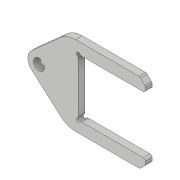
# Autodesk Inventor part: FRC003-1
Saved by Autodesk Inventor 2020 (Build 240168000, 168)
## iProperties
Created: 2020-02-07
Part Number: FRC003-1
Material: Generic
Document SubType Name: Modeling
Designer: Juan Carlos Botero
Density: 1 g/cm^3
Appearance: Default
Mass: 6.52409 g
Surface Area: 32.0611 cm^2
Volume: 6.52409 cm^3
Author: Juan Carlos Botero
Title: SOPORTE PIVOTE
Autodesk Inventor part; units mm, degrees
ref_plane "YZ Plane" through (0, 0, 0) normal (1, 0, 0) x (0, 1, 0)
ref_plane "XZ Plane" through (0, 0, 0) normal (0, 1, 0) x (-1, 0, 0)
ref_plane "XY Plane" through (0, 0, 0) normal (0, 0, 1) x (1, 0, 0)
sketch "Sketch1" plane through (0, 0, 0) normal (0, 0, 1) x (1, 0, 0)
  circle A0 centre (-790.1228, -10.9134) radius 9.525 projected
  ellipse E0 centre (61.5218, 18.65) end of major axis (52.5416, 18.65) minor radius 6.35 (61.5218, 25) -> (52.5416, 18.65) ccw
  line L0 (61.5218, 25) -> (114.272, 25)
  ellipse E1 centre (114.272, 18.65) end of major axis (105.2917, 18.65) minor radius 6.35 (123.2522, 18.65) -> (114.272, 25) ccw
  line L1 (123.2522, 18.65) -> (123.2522, -18.65)
  ellipse E2 centre (114.272, -18.65) end of major axis (105.2917, -18.65) minor radius 6.35 (114.272, -25) -> (123.2522, -18.65) ccw
  line L2 (114.272, -25) -> (61.5218, -25)
  ellipse E3 centre (61.5218, -18.65) end of major axis (52.5416, -18.65) minor radius 6.35 (52.5416, -18.65) -> (61.5218, -25) ccw
  line L3 (52.5416, -18.65) -> (52.5416, 18.65)
  line L4 (114.272, 21.825) -> (61.5218, 21.825)
  ellipse E4 centre (61.5218, 18.65) end of major axis (57.0317, 18.65) minor radius 3.175 (61.5218, 21.825) -> (57.0317, 18.65) ccw
  line L5 (57.0317, 18.65) -> (57.0317, -18.65)
  ellipse E5 centre (61.5218, -18.65) end of major axis (57.0317, -18.65) minor radius 3.175 (57.0317, -18.65) -> (61.5218, -21.825) ccw
  line L6 (61.5218, -21.825) -> (114.272, -21.825)
  ellipse E6 centre (114.272, -18.65) end of major axis (109.7818, -18.65) minor radius 3.175 (114.272, -21.825) -> (118.7621, -18.65) ccw
  line L7 (118.7621, -18.65) -> (118.7621, 18.65)
  ellipse E7 centre (114.272, 18.65) end of major axis (109.7818, 18.65) minor radius 3.175 (118.7621, 18.65) -> (114.272, 21.825) ccw
  circle A1 centre (17.6912, 0) radius 5 projected
  circle A2 centre (17.6912, 0) radius 10
  line L8 (15.357, 9.7238) -> (52.5416, 18.65)
  line L9 (52.5416, -18.65) -> (15.357, -9.7238)
  dimension "d4" = 20
  constraints: 20 end point, 4 horizontal, 4 vertical, 2 point on circle, 2 tangent, 1 centre point, 1 coincident, 56 other
  measures "d4" diameter of A2
extrude "Extrusion1" add sketch "Sketch1" along normal blind 6 contours L3 L9 A2 L8 | A2
chamfer "Chamfer1" distance 5 angle 45 1 edges at (52.5416, 0, 6)
thicken "Thicken1" operation add thickness 3 both sides no extend neighbours yes toward (-0.7071068, 0, -0.7071068) faces at (50.8749, 5.8166, 2.6667)
sketch "Sketch2" plane through (0, 0, 0) normal (0, 0, -1) x (-1, 0, 0)
  line L0 (-49.2989, -17.8716) -> (-49.2989, 17.8716) projected
  line L1 (-15.357, -9.7238) -> (-49.2989, -17.8716) projected
  arc A0 (-15.357, -9.7238) -> (-15.357, 9.7238) centre (-17.6912, 0) ccw projected
  line L2 (-49.2989, 17.8716) -> (-15.357, 9.7238) projected
  circle A1 centre (-17.6912, 0) radius 5 projected
  line L3 (-112.6912, -35.5) -> (-42.6912, -35.5)
  line L4 (-42.6912, -35.5) -> (-42.6912, 35.5)
  line L5 (-42.6912, 35.5) -> (-112.6912, 35.5)
  line L6 (-112.6912, -35.5) -> (-42.6912, 35.5) construction
  line L7 (-42.6912, -35.5) -> (-112.6912, 35.5) construction
  line L8 (-42.6912, 35.5) -> (-11.061, 7.486)
  arc A2 (-15.357, -9.7238) -> (-15.357, 9.7238) centre (-17.6912, 0) ccw projected
  line L9 (-42.6912, -35.5) -> (-11.061, -7.486)
  line L10 (-102.6912, -25.5) -> (-52.6912, -25.5)
  line L11 (-52.6912, -25.5) -> (-52.6912, 25.5)
  line L12 (-52.6912, 25.5) -> (-102.6912, 25.5)
  line L13 (-102.6912, -25.5) -> (-52.6912, 25.5) construction
  line L14 (-52.6912, -25.5) -> (-102.6912, 25.5) construction
  line L15 (-102.6912, 25.5) -> (-112.6912, 25.5)
  line L16 (-112.6912, -25.5) -> (-102.6912, -25.5)
  line L17 (-112.6912, 35.5) -> (-112.6912, 25.5)
  line L18 (-112.6912, -25.5) -> (-112.6912, -35.5)
  line L19 (-49.2989, -17.8716) -> (-49.2989, 17.8716) projected
  point P0 (0, 0)
  point P1 (-77.6912, 0)
  point P2 (-49.2989, 0)
  point P3 (-77.6912, 0)
  point P4 (-11.061, -7.486)
  point P5 (-11.061, 7.486)
  point P6 (-49.2989, 0)
  point P7 (-52.6912, 0)
  dimension "d13" = 51
  dimension "d14" = 35
  dimension "d15" = 10
  dimension "d16" = 50
  dimension "d17" = 10
  dimension "d30" = 71
  constraints: 32 end point, 8 midpoint, 3 horizontal, 2 horizontal alignment, 2 parallel, 2 perpendicular, 2 point on circle, 2 tangent, 2 vertical, 1 collinear, 1 vertical alignment
  measures "d13" distance of L11.end L10.end
  measures "d14" distance from line of A0.centre L11
  measures "d15" distance between parallel lines of L12 L5
  measures "d16" distance of L11.end L12.end
  measures "d17" distance between parallel lines of L4 L11
  measures "d30" distance between parallel lines of L3 L5
extrude "Extrusion2" add sketch "Sketch2" against normal up to surface (6 mm away)
chamfer "Chamfer2" distance 5 angle 45 2 edges at (112.6912, 35.5, 3) (112.6912, -35.5, 3)
sketch "Sketch3" plane through (0, 0, 0) normal (0, 0, -1) x (-1, 0, 0)
  line L0 (-107.6912, -35.5) -> (-112.6912, -30.5) projected
  line L1 (-107.6912, -35.5) -> (-42.6912, -35.5) projected
  line L2 (-42.6912, -35.5) -> (-11.061, -7.486) projected
  arc A0 (-11.061, -7.486) -> (-11.061, 7.486) centre (-17.6912, 0) ccw projected
  line L3 (-11.061, 7.486) -> (-42.6912, 35.5) projected
  line L4 (-42.6912, 35.5) -> (-107.6912, 35.5) projected
  line L5 (-112.6912, 30.5) -> (-107.6912, 35.5) projected
  line L6 (-112.6912, 30.5) -> (-112.6912, 25.5) projected
  line L7 (-112.6912, 25.5) -> (-52.6912, 25.5) projected
  line L8 (-52.6912, 25.5) -> (-52.6912, -25.5) projected
  line L9 (-52.6912, -25.5) -> (-112.6912, -25.5) projected
  line L10 (-112.6912, -25.5) -> (-112.6912, -30.5) projected
  circle A1 centre (-17.6912, 0) radius 5 projected
  line L11 (-52.6912, 25.5) -> (-52.6912, -25.5) projected
  circle A2 centre (-52.6912, 25.5) radius 1.5
  circle A3 centre (-52.6912, -25.5) radius 1.5
  point P0 (0, 0)
  dimension "d23" = 3
  dimension "d24" = 3
  constraints: 2 centre point, 2 coincident
  measures "d23" diameter of A2
  measures "d24" diameter of A3
extrude "Extrusion3" cut sketch "Sketch3" against normal through all contours A3 L8 L9 | L9 L8 A3 | A2 L7 L8 | L8 L7 A2
fillet "Fillet1" radius 2 4 edges at (52.6912, -24, 3) (54.1912, -25.5, 3) (54.1912, 25.5, 3) (52.6912, 24, 3)
fillet "Fillet2" radius 2 6 edges at (107.6912, -35.5, 3) (112.6912, -30.5, 3) (107.6912, 35.5, 3) (112.6912, 30.5, 3) (112.6912, 25.5, 3) (112.6912, -25.5, 3)
fillet "Fillet3" radius 20 2 edges at (42.6912, 35.5, 3) (42.6912, -35.5, 3)
body "Solid1"
